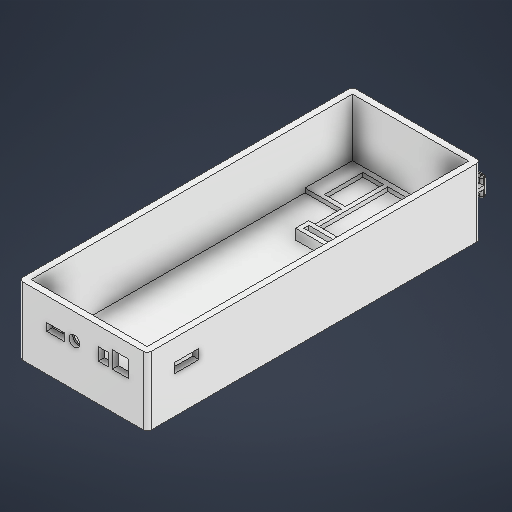
# Autodesk Inventor part: module_command
Saved by Autodesk Inventor 2025.4 (Build 294407000, 407)
## iProperties
Created: 2025-09-05
Part Number: module_command
Material: PC/ABS Plastic
Document SubType Name: Modeling
Designer: sam
Density: 1.1 g/cm^3
Appearance: Smooth - White
Author: sam
Autodesk Inventor part; units mm, degrees
ref_plane "YZ Plane" through (0, 0, 0) normal (1, 0, 0) x (0, 1, 0)
ref_plane "XZ Plane" through (0, 0, 0) normal (0, 1, 0) x (-1, 0, 0)
ref_plane "XY Plane" through (0, 0, 0) normal (0, 0, 1) x (1, 0, 0)
sketch "Sketch1" plane through (0, 0, 0) normal (0, 1, 0) x (-1, 0, 0)
  line L0 (-31.2, -81) -> (31.2, -81)
  line L1 (31.2, -81) -> (31.2, 81)
  line L2 (31.2, 81) -> (-31.2, 81)
  line L3 (-31.2, 81) -> (-31.2, -81)
  line L4 (-31.2, -81) -> (31.2, 81) construction
  line L5 (31.2, -81) -> (-31.2, 81) construction
  point P0 (0, 0)
  dimension "d0" = 62.4
  dimension "d1" = 162
  constraints: 12 end point, 2 midpoint, 2 parallel, 1 horizontal, 1 perpendicular
  measures "d0" distance of L2.end L1.end
  measures "d1" distance of L1.end L0.end
extrude "Extrusion1" add sketch "Sketch1" along normal blind 3
sketch "Sketch2" plane through (0, 3, 0) normal (0, 1, 0) x (1, 0, 0)
  line L0 (-31.2, 81) -> (-31.2, -81) projected
  line L1 (-31.2, -81) -> (31.2, -81) projected
  line L2 (31.2, -81) -> (31.2, 81) projected
  line L3 (31.2, 81) -> (-31.2, 81) projected
  line L4 (31.2, 81) -> (-31.2, 81)
  line L5 (-31.2, 81) -> (-31.2, -81)
  line L6 (-31.2, -81) -> (31.2, -81)
  line L7 (31.2, -81) -> (31.2, 81)
  line L8 (31.2, 81) -> (-31.2, -81) construction
  line L9 (-31.2, 81) -> (31.2, -81) construction
  line L10 (28.2, 78) -> (-28.2, 78)
  line L11 (-28.2, 78) -> (-28.2, -78)
  line L12 (-28.2, -78) -> (28.2, -78)
  line L13 (28.2, -78) -> (28.2, 78)
  line L14 (28.2, 78) -> (-28.2, -78) construction
  line L15 (-28.2, 78) -> (28.2, -78) construction
  point P0 (0, 0)
  dimension "d4" = 0
  dimension "d5" = 0
  dimension "d6" = 3
  dimension "d7" = 3
  constraints: 24 end point, 4 midpoint, 4 parallel, 2 horizontal, 2 perpendicular
  measures "d4" distance between parallel lines of L0 L5
  measures "d5" distance between parallel lines of L1 L6
  measures "d6" distance between parallel lines of L5 L11
  measures "d7" distance between parallel lines of L6 L12
extrude "Extrusion2" add sketch "Sketch2" along normal blind 30
fillet "Fillet1" radius 2 4 edges at (31.2, 16.5, 81) (31.2, 16.5, -81) (-31.2, 16.5, 81) (-31.2, 16.5, -81)
sketch "Sketch9" plane through (0, 3, 0) normal (0, 1, 0) x (1, 0, 0)
  line L0 (28.2, 78) -> (-28.2, 78) projected
  line L1 (-28.2, 78) -> (-28.2, -78) projected
  line L2 (-28.2, -78) -> (28.2, -78) projected
  line L3 (28.2, -78) -> (28.2, 78) projected
  line L4 (-28.2, -75.6) -> (28.2, -75.6)
  line L5 (28.2, -75.6) -> (28.2, -73.6)
  line L6 (28.2, -73.6) -> (-28.2, -73.6)
  line L7 (-28.2, -73.6) -> (-28.2, -75.6)
  line L8 (-28.2, 78) -> (-28.2, -78) projected
  line L9 (-28.2, 32.8) -> (28.2, 32.8)
  line L10 (28.2, 32.8) -> (28.2, 34.8)
  line L11 (28.2, 34.8) -> (-28.2, 34.8)
  line L12 (-28.2, 34.8) -> (-28.2, 32.8)
  line L13 (-28.2, 34.8) -> (-10.6, 34.8)
  line L14 (-10.6, 34.8) -> (-10.6, 32.8)
  line L15 (-10.6, 32.8) -> (-28.2, 32.8)
  line L16 (-28.2, 32.8) -> (-28.2, 34.8)
  line L17 (28.2, 39.2) -> (-10.6, 39.2)
  line L18 (-10.6, 39.2) -> (-10.6, 37.2)
  line L19 (-10.6, 37.2) -> (28.2, 37.2)
  line L20 (28.2, 37.2) -> (28.2, 39.2)
  line L21 (-10.6, 37.2) -> (-8.6, 37.2)
  line L22 (-8.6, 37.2) -> (-8.6, 34.8)
  line L23 (-8.6, 34.8) -> (-10.6, 34.8)
  line L24 (-10.6, 34.8) -> (-10.6, 37.2)
  point P0 (0, 0)
  point P1 (28.2, 14.2)
  point P2 (-28.2, 34.8)
  point P3 (28.2, 32.8)
  point P4 (-28.2, -73.6)
  point P5 (28.2, -75.6)
  point P6 (-10.6, 34.8)
  point P7 (28.2, 37.2)
  dimension "d79" = 2
  dimension "d80" = 2.4
  dimension "d81" = 2
  dimension "d82" = 106.4
  dimension "d87" = 17.6
  dimension "d163" = 2
  dimension "d164" = 2.4
  dimension "d165" = 17.6
  dimension "d166" = 2
  constraints: 40 end point, 10 parallel, 8 point on line, 5 horizontal, 5 perpendicular
  measures "d79" distance of L5.end L4.end
  measures "d80" distance between parallel lines of L2 L4
  measures "d81" distance of L10.end L9.end
  measures "d82" distance between parallel lines of L6 L9
  measures "d87" distance of L14.end L15.end
  measures "d163" distance between parallel lines of L17 L19
  measures "d164" distance between parallel lines of L11 L19
  measures "d165" distance between parallel lines of L8 L18
  measures "d166" distance of L22.end L23.end
extrude "Extrusion9" add sketch "Sketch9" along normal blind 5 contours L3 L19 L18 L17 | L24 L19 L22 L11 | L11 L3 L9 L14 | L6 L3 L4 L1
sketch "Sketch10" plane through (0, 3, 0) normal (0, 1, 0) x (1, 0, 0)
  line L0 (-28.2, -73.6) -> (28.2, -73.6) projected
  line L1 (28.2, -73.6) -> (28.2, 32.8) projected
  line L2 (28.2, 32.8) -> (-10.6, 32.8) projected
  line L3 (-8.6, 34.8) -> (28.2, 34.8) projected
  line L4 (28.2, 34.8) -> (28.2, 37.2) projected
  line L5 (28.2, 78) -> (-28.2, 78) projected
  line L6 (-28.2, 78) -> (-28.2, -73.6) projected
  line L7 (-28.2, 37.2) -> (28.2, 37.2)
  line L8 (-28.2, 70.4) -> (-28.2, 37.2)
  line L9 (-28.2, 37.2) -> (28.2, 37.2)
  line L10 (28.2, 37.2) -> (28.2, 39.2)
  line L11 (28.2, 39.2) -> (-28.2, 39.2)
  line L12 (-28.2, 39.2) -> (-28.2, 37.2)
  line L13 (28.2, 34.8) -> (28.2, 78) projected
  line L14 (-28.2, 39.2) -> (28.2, 39.2)
  line L15 (28.2, 39.2) -> (28.2, 75.6)
  line L16 (28.2, 75.6) -> (-22.2, 75.6)
  line L17 (-22.2, 75.6) -> (28.2, 75.6)
  line L18 (28.2, 75.6) -> (28.2, 68)
  line L19 (-22.2, 73.6) -> (-22.2, 75.6)
  line L20 (28.2, 39.2) -> (26.2, 39.2)
  line L21 (26.2, 39.2) -> (26.2, 75.6)
  line L22 (26.2, 75.6) -> (28.2, 75.6)
  line L23 (28.2, 75.6) -> (28.2, 39.2)
  line L24 (26.2, 39.2) -> (9.8, 39.2)
  line L25 (9.8, 39.2) -> (9.8, 75.6)
  line L26 (9.8, 75.6) -> (26.2, 75.6)
  line L27 (26.2, 75.6) -> (26.2, 39.2)
  line L28 (9.8, 39.2) -> (7.8, 39.2)
  line L29 (7.8, 39.2) -> (7.8, 75.6)
  line L30 (7.8, 75.6) -> (9.8, 75.6)
  line L31 (9.8, 75.6) -> (9.8, 39.2)
  line L32 (7.8, 39.2) -> (-8.6, 39.2)
  line L33 (-8.6, 39.2) -> (-8.6, 75.6)
  line L34 (-8.6, 75.6) -> (7.8, 75.6)
  line L35 (7.8, 75.6) -> (7.8, 39.2)
  line L36 (-8.6, 39.2) -> (-10.6, 39.2)
  line L37 (-10.6, 39.2) -> (-10.6, 75.6)
  line L38 (-10.6, 75.6) -> (-8.6, 75.6)
  line L39 (-8.6, 75.6) -> (-8.6, 39.2)
  line L40 (-22.2, 75.6) -> (-20.7, 75.6)
  line L41 (-20.7, 75.6) -> (-20.7, 39.2)
  line L42 (-20.7, 39.2) -> (-22.2, 39.2)
  line L43 (-22.2, 39.2) -> (-22.2, 75.6)
  line L44 (-10.6, 39.2) -> (-10.6, 57)
  line L45 (-10.6, 57) -> (-20.7, 57)
  line L46 (-20.7, 57) -> (-20.7, 39.2)
  line L47 (-10.6, 39.2) -> (28.2, 39.2) projected
  line L48 (28.2, 39.2) -> (28.2, 78) projected
  line L49 (-10.6, 32.8) -> (-10.6, 39.2) projected
  line L50 (28.2, 37.2) -> (-8.6, 37.2) projected
  line L51 (-8.6, 37.2) -> (-8.6, 34.8) projected
  line L52 (28.2, -75.6) -> (-28.2, -75.6) projected
  line L53 (-28.2, -75.6) -> (-28.2, -78) projected
  line L54 (-28.2, -78) -> (28.2, -78) projected
  line L55 (28.2, -78) -> (28.2, -75.6) projected
  line L56 (-10.6, 39.2) -> (-10.6, 37.2)
  line L57 (-10.6, 55) -> (-22.2, 55)
  line L58 (-10.6, 39.2) -> (-10.6, 39.2)
  line L59 (-10.6, 39.2) -> (-10.6, 32.8)
  line L60 (-10.6, 32.8) -> (-10.6, 32.8)
  line L61 (-10.6, 32.8) -> (-10.6, 39.2)
  line L62 (-22.2, 55) -> (-28.2, 55)
  point P0 (0, 0)
  point P1 (28.2, 37.2)
  point P2 (7.8, 39.2)
  point P3 (-8.6, 39.2)
  point P4 (-10.6, 39.2)
  point P5 (26.2, 39.2)
  point P6 (9.8, 39.2)
  point P7 (28.2, 37.2)
  point P8 (-10.6, 37.2)
  point P9 (28.2, 39.2)
  point P10 (-25.2, 72.6)
  point P11 (-10.6, 75.6)
  point P12 (-10.6, 37.2)
  point P13 (-10.6, 39.2)
  point P14 (-10.6, 55)
  point P15 (-20.7, 75.6)
  point P16 (-25.2, 52)
  point P17 (-10.6, 37.2)
  point P18 (-28.2, 39.2)
  point P19 (-10.6, 39.2)
  point P20 (-10.6, 37.2)
  point P21 (-10.6, 39.2)
  point P22 (-10.6, 39.2)
  point P23 (-20.7, 55)
  point P24 (-10.6, 39.2)
  point P25 (-10.1, 32.8)
  point P26 (28.2, 39.2)
  point P27 (-10.6, 39.2)
  point P28 (-8.6, 39.2)
  point P29 (28.2, 39.2)
  point P30 (-10.6, 32.8)
  point P31 (-10.1, 39.2)
  point P32 (-10.1, 39.2)
  dimension "d90" = 2
  dimension "d91" = 36.4
  dimension "d93" = 2
  dimension "d94" = 16.4
  dimension "d95" = 2
  dimension "d96" = 16.4
  dimension "d97" = 2
  dimension "d98" = 1.5
  dimension "d167" = 2.4
  dimension "d172" = 18.6
  dimension "d173" = 2
  constraints: 92 end point, 18 parallel, 15 point on line, 12 perpendicular, 11 horizontal, 1 collinear
  measures "d90" distance of L10.end L9.end
  measures "d91" distance of L15.end L14.end
  measures "d93" distance of L21.end L22.end
  measures "d94" distance of L25.end L26.end
  measures "d95" distance of L29.end L30.end
  measures "d96" distance of L33.end L34.end
  measures "d97" distance of L37.end L38.end
  measures "d98" distance of L41.end L42.end
  measures "d167" distance between parallel lines of L5 L16
  measures "d172" distance between parallel lines of L16 L45
  measures "d173" distance between parallel lines of L45 L57
extrude "Extrusion10" add sketch "Sketch10" along normal blind 2 contours L6 L5 L13 L16 L19 L43 L62 | L37 L16 L33 L11 | L43 L19 L16 L41 L57 | L57 L41 L45 L37 | L11 L21 L16 L13 | L29 L16 L25 L11
sketch "Sketch11" plane through (-23.2, 5, 81) normal (0, 0, 1) x (1, 0, 0)
  line L0 (-6, 28) -> (52.4, 28) projected
  line L1 (5.5, 13) -> (14.2, 13)
  line L2 (14.2, 13) -> (14.2, 16.7)
  line L3 (14.2, 16.7) -> (5.5, 16.7)
  line L4 (5.5, 16.7) -> (5.5, 13)
  line L5 (45.4, 13) -> (37.34, 13)
  line L6 (37.34, 13) -> (37.34, 21.2)
  line L7 (37.34, 21.2) -> (45.4, 21.2)
  line L8 (45.4, 21.2) -> (45.4, 13)
  circle A0 centre (19, 15.6) radius 2.6
  line L9 (48.4, 0) -> (48.4, 30) projected
  line L10 (52.4, 28) -> (52.4, -5) projected
  line L11 (-6, -5) -> (-6, 28) projected
  line L12 (-6, -5) -> (52.4, -5) projected
  line L13 (54.4, -5) -> (54.4, 28) projected
  line L14 (-8, 28) -> (-8, -5) projected
  line L15 (30.64, 13) -> (35.34, 13)
  line L16 (35.34, 13) -> (35.34, 19.1)
  line L17 (35.34, 19.1) -> (30.64, 19.1)
  line L18 (30.64, 19.1) -> (30.64, 13)
  point P0 (23.2, -5)
  point P1 (46.4, 0)
  point P2 (0, 0)
  dimension "d110" = 8.7
  dimension "d111" = 3.7
  dimension "d112" = 8.06
  dimension "d113" = 8.2
  dimension "d114" = 5.2
  dimension "d149" = 9
  dimension "d150" = 13.5
  dimension "d151" = 27
  dimension "d152" = 18
  dimension "d153" = 18
  dimension "d154" = 18
  dimension "d168" = 4.7
  dimension "d169" = 6.1
  dimension "d170" = 2
  dimension "d171" = 18
  constraints: 24 end point, 6 parallel, 3 horizontal, 3 perpendicular, 1 centre point
  measures "d110" distance of L3.end L2.end
  measures "d111" distance of L2.end L1.end
  measures "d112" distance of L6.end L7.end
  measures "d113" distance of L5.end L6.end
  measures "d114" diameter of A0
  measures "d149" distance between parallel lines of L8 L13
  measures "d150" distance between parallel lines of L14 L4
  measures "d151" distance from line of A0.centre L14
  measures "d152" distance between parallel lines of L12 L5
  measures "d153" distance between parallel lines of L12 L1
  measures "d154" distance edge to line of A0 L12
  measures "d168" distance of L17.end L16.end
  measures "d169" distance of L16.end L15.end
  measures "d170" distance between parallel lines of L6 L16
  measures "d171" distance between parallel lines of L12 L15
extrude "Extrusion11" cut sketch "Sketch11" against normal blind 3 contours L4 L3 L2 L1 | L5 L6 L7 L8 | A0 | L18 L17 L16 L15
sketch "Sketch12" plane through (28.2, 3, 78) normal (0, 0, -1) x (-1, 0, 0)
  line L0 (14.06, 23.2) -> (14.06, 15) projected
  line L1 (14.06, 15) -> (6, 15) projected
  line L2 (6, 15) -> (6, 23.2) projected
  line L3 (6, 23.2) -> (14.06, 23.2) projected
  line L4 (37.2, 18.7) -> (45.9, 18.7) projected
  line L5 (45.9, 18.7) -> (45.9, 15) projected
  line L6 (45.9, 15) -> (37.2, 15) projected
  line L7 (37.2, 15) -> (37.2, 18.7) projected
  circle A0 centre (32.4, 17.6) radius 2.6 projected
  line L8 (56.4, 0) -> (0, 0) projected
  line L9 (56.4, 0) -> (56.4, 30) projected
  line L10 (0, 30) -> (56.4, 30) projected
  line L11 (0, 0) -> (0, 30) projected
  circle A1 centre (32.4, 17.6) radius 3.05
  point P0 (28.2, -3)
  dimension "d128" = 6.1
  constraints: 1 centre point, 1 coincident
  measures "d128" diameter of A1
extrude "Extrusion12" cut sketch "Sketch12" against normal blind 1.2 contours A1
sketch "Sketch13" plane through (23.2, 5, -81) normal (0, 0, -1) x (-1, 0, 0)
  line L0 (-5, 18) -> (51.4, 18)
  line L1 (51.4, 18) -> (51.4, 8.4)
  line L2 (51.4, 8.4) -> (-5, 8.4)
  line L3 (-5, 8.4) -> (-5, 18)
  line L4 (54.4, -5) -> (54.4, 28) projected
  line L5 (-8, 28) -> (-8, -5) projected
  line L6 (-6, -5) -> (52.4, -5) projected
  point P0 (23.2, -5)
  point P1 (51.4, 0)
  point P2 (-5, 0)
  point P3 (-8, -5)
  point P4 (54.4, 11.5)
  point P5 (51.4, 13.2)
  dimension "d131" = 9.6
  dimension "d146" = 3
  dimension "d147" = 3
  dimension "d156" = 23
  constraints: 8 end point, 2 parallel, 1 horizontal, 1 midpoint, 1 perpendicular, 3 other
  measures "d131" distance of L0.end L1.end
  measures "d156" distance between parallel lines of L0 L6
extrude "Extrusion13" add sketch "Sketch13" along normal blind 6
sketch "Sketch14" plane through (-28.2, 13.4, -81) normal (-1, 0, 0) x (0, 0, 1)
  line L0 (0, 9.6) -> (0, 0) projected
  line L1 (0, 9.6) -> (-6, 9.6) projected
  line L2 (-6, 0) -> (-6, 9.6) projected
  line L3 (0, 0) -> (-6, 0) projected
  line L4 (0, 9.6) -> (-3.4, 9.6)
  line L5 (-3.4, 9.6) -> (-3.4, 6.6)
  line L6 (-3.4, 6.6) -> (0, 6.6)
  line L7 (0, 6.6) -> (0, 9.6)
  line L8 (0, 0) -> (-3.4, 0)
  line L9 (-3.4, 0) -> (-3.4, 3)
  line L10 (-3.4, 3) -> (0, 3)
  line L11 (0, 3) -> (0, 0)
  point P0 (81, -13.4)
  point P1 (0, 6.6)
  dimension "d137" = 3.4
  dimension "d138" = 3
  dimension "d139" = 3.4
  dimension "d140" = 3
  constraints: 16 end point, 4 parallel, 2 horizontal, 2 perpendicular
  measures "d137" distance of L6.end L5.end
  measures "d138" distance of L5.end L4.end
  measures "d139" distance of L9.end L10.end
  measures "d140" distance of L8.end L9.end
extrude "Extrusion14" cut sketch "Sketch14" against normal up to surface (56.4 mm away) contours L0 L6 L5 L1 | L0 L3 L9 L10
fillet "Fillet5" radius 1 18 edges at (0, 23, -87) (0, 23, -84.4) (0, 13.4, -87) (0, 13.4, -84.4) (-28.2, 16.4, -82.7) (-28.2, 20, -82.7) (28.2, 16.4, -82.7) (28.2, 20, -82.7) (-28.2, 18.2, -87) (-28.2, 21.5, -84.4) (-28.2, 14.9, -84.4) (-28.2, 23, -85.7) (-28.2, 13.4, -85.7) (28.2, 23, -85.7) (28.2, 13.4, -85.7) (28.2, 14.9, -84.4) (28.2, 18.2, -87) (28.2, 21.5, -84.4)
sketch "Sketch15" plane through (31.2, 0, 79) normal (1, 0, 0) x (0, 0, -1)
  line L0 (11, 22.7) -> (23.1, 22.7)
  line L1 (23.1, 22.7) -> (23.1, 18)
  line L2 (23.1, 18) -> (11, 18)
  line L3 (11, 18) -> (11, 22.7)
  line L4 (-2, 33) -> (-2, 0) projected
  line L5 (0, 0) -> (158, 0) projected
  point P0 (79, 0)
  dimension "d157" = 12.1
  dimension "d158" = 4.7
  dimension "d159" = 13
  dimension "d160" = 18
  constraints: 8 end point, 2 parallel, 1 horizontal, 1 perpendicular
  measures "d157" distance of L1.end L2.end
  measures "d158" distance of L0.end L1.end
  measures "d159" distance between parallel lines of L4 L3
  measures "d160" distance between parallel lines of L5 L2
extrude "Extrusion15" cut sketch "Sketch15" against normal blind 3
body "Solid1"
